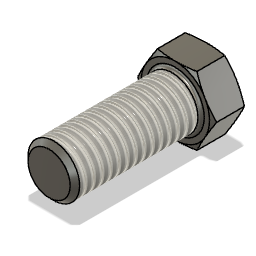
bolt v4 (Autodesk Fusion 360 design; units mm, degrees)
Autodesk Fusion 360 part; units mm, degrees
sketch "草图1" plane through (0, 0, 0) normal (0, 0, 1) x (1, 0, 0) in component "Component"
  line L0 (1.875, 3.2476) -> (3.75, 0)
  line L1 (-1.875, 3.2476) -> (1.875, 3.2476)
  line L2 (-3.75, 0) -> (-1.875, 3.2476)
  line L3 (-1.875, -3.2476) -> (-3.75, 0)
  line L4 (1.875, -3.2476) -> (-1.875, -3.2476)
  line L5 (3.75, 0) -> (1.875, -3.2476)
extrude "拉伸1" add sketch "草图1" along normal blind 3 in component "Component"
sketch "草图2" plane through (0, 0, 0) normal (0, 0, 1) x (1, 0, 0) in component "Component"
  circle A0 centre (0, 0) radius 2.5
extrude "拉伸2" add sketch "草图2" along normal blind 15 in component "Component"
chamfer "倒角1" distance 0.5 angle 45 1 edges at (-2.3308, -0.904, 15) in component "Component"
fillet "圆角1" radius 0.3 1 edges at (-2.3308, 0.904, 3) in component "Component"
sketch "草图3" plane through (0, 0, 0) normal (0, 1, 0) x (1, 0, 0) in component "Component"
  line L0 (3.2476, 0) -> (3.75, 0)
  line L1 (3.75, 0) -> (3.75, -0.1829)
  line L2 (3.75, -0.1829) -> (3.2476, 0)
  line L3 (3.2476, -3) -> (3.75, -3)
  line L4 (3.75, -3) -> (3.75, -2.8171)
  line L5 (3.75, -2.8171) -> (3.2476, -3)
revolve "旋转1" cut sketch "草图3" angle 360 about axis through (0, 0, 1.75) along (0, 0, 1) contours L3 L4 L5 in component "Component"
revolve "旋转2" cut sketch "草图3" angle 360 about axis through (0, 0, 1.75) along (0, 0, 1) contours L0 L1 L2 in component "Component"
thread "螺纹1" "ISO Metric profile 5.0 M5x0.8 6g" major diameter 4.901 minor diameter 3.9895 pitch 0.8 angle 60 resizes the face on face at (2.4969, -0.1246, 10.7667) in component "Component"
component "Component" placed x (1, 0, 0) y (0, 1, 0) z (0, 0, 1) at (0, 0, 0)
named bodies: "Bolt"
